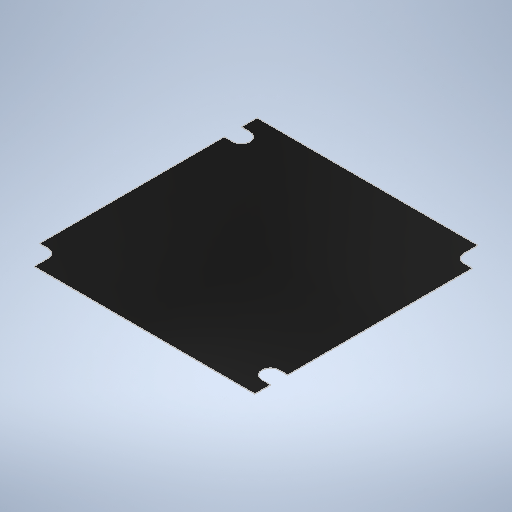
# Autodesk Inventor part: Coverplate Film
Saved by Autodesk Inventor 2025 (Build 290162000, 162)
## iProperties
Created: 2022-02-23
Part Number: Coverplate Film
Material: Thermoplastic Resin
Document SubType Name: Modeling
Designer: Caleb
Density: 1.28 g/cm^3
Appearance: Smooth - Black
Author: Caleb
Autodesk Inventor part; units mm, degrees
ref_plane "YZ Plane" through (0, 0, 0) normal (1, 0, 0) x (0, 1, 0)
ref_plane "XZ Plane" through (0, 0, 0) normal (0, 1, 0) x (-1, 0, 0)
ref_plane "XY Plane" through (0, 0, 0) normal (0, 0, 1) x (1, 0, 0)
sketch "Sketch1" plane through (0, 0, 0) normal (0, 1, 0) x (-1, 0, 0)
  line L0 (-20.8, -21) -> (20.8, -21)
  line L1 (20.8, -21) -> (20.8, 21)
  line L2 (20.8, 21) -> (-20.8, 21)
  line L3 (-20.8, 21) -> (-20.8, -21)
  line L4 (-20.8, -21) -> (20.8, 21) construction
  line L5 (20.8, -21) -> (-20.8, 21) construction
  point P0 (0, 0)
  dimension "d0" = 42
  dimension "d1" = 41.6
  constraints: 12 end point, 2 midpoint, 2 parallel, 1 horizontal, 1 perpendicular
  measures "d0" distance of L0.end L1.end
  measures "d1" distance of L1.end L2.end
extrude "Extrusion1" add sketch "Sketch1" along normal blind 0.08
sketch "Sketch2" plane through (0, 0.08, 0) normal (0, 1, 0) x (1, 0, 0)
  line L0 (-20.8, 21) -> (-20.8, -21) projected
  line L1 (-20.8, 18.3058) -> (-20.8, 15.1942)
  line L2 (-20.8, -17.05) -> (-20.8, -20.05)
  line L3 (20.8, 21) -> (-20.8, 21) projected
  line L4 (-22.3, 16.75) -> (-19.3, 16.75) construction
  line L5 (-22.3, 15.25) -> (-19.3, 15.25)
  line L6 (-19.3, 18.25) -> (-22.3, 18.25)
  arc A0 (-22.3, 18.25) -> (-22.3, 15.25) centre (-22.3, 16.75) ccw
  arc A1 (-19.3, 15.25) -> (-19.3, 18.25) centre (-19.3, 16.75) ccw
  line L7 (-22.3, -18.55) -> (-19.3, -18.55) construction
  line L8 (-22.3, -20.05) -> (-19.3, -20.05)
  line L9 (-19.3, -17.05) -> (-22.3, -17.05)
  arc A2 (-22.3, -17.05) -> (-22.3, -20.05) centre (-22.3, -18.55) ccw
  arc A3 (-19.3, -20.05) -> (-19.3, -17.05) centre (-19.3, -18.55) ccw
  line L10 (-20.8, -21) -> (20.8, -21) projected
  line L11 (20.8, -21) -> (20.8, 21) projected
  line L12 (22.3, -16.75) -> (19.3, -16.75) construction
  line L13 (22.3, -15.25) -> (19.3, -15.25)
  line L14 (20.8, -18.3058) -> (20.8, -15.1942)
  arc A4 (22.3, -18.25) -> (22.3, -15.25) centre (22.3, -16.75) ccw
  arc A5 (19.3, -15.25) -> (19.3, -18.25) centre (19.3, -16.75) ccw
  line L15 (19.3, -18.25) -> (22.3, -18.25)
  arc A6 (19.3, 20.05) -> (19.3, 17.05) centre (19.3, 18.55) ccw
  line L16 (19.3, 17.05) -> (22.3, 17.05)
  line L17 (20.8, 17.05) -> (20.8, 20.05)
  line L18 (22.3, 18.55) -> (19.3, 18.55) construction
  line L19 (22.3, 20.05) -> (19.3, 20.05)
  arc A7 (22.3, 17.05) -> (22.3, 20.05) centre (22.3, 18.55) ccw
  point P0 (-20.8, 16.75)
  point P1 (-20.8, 16.75)
  point P2 (-20.8, -18.55)
  point P3 (0, 0)
  point P4 (20.8, -16.75)
  point P5 (20.8, -16.75)
  point P6 (20.8, 18.55)
  point P7 (20.8, 17.05)
  point P8 (20.8, -18.25)
  point P9 (20.8, -15.25)
  point P10 (-20.8, 18.25)
  point P11 (-20.8, 15.25)
  dimension "d16" = 1.5
  dimension "d17" = 4.25
  dimension "d18" = 1.5
  dimension "d20" = 1.5
  dimension "d22" = 39.55
  dimension "d23" = 21
  dimension "d24" = 42
  dimension "d25" = 41.6
  dimension "d26" = 20.8
  dimension "d29" = 360
  constraints: 40 end point, 16 point on circle, 8 centre point, 8 tangent, 5 point on line, 3 midpoint, 2 collinear, 2 horizontal, 2 parallel, 1 horizontal alignment, 1 vertical alignment, 63 other
  measures "d16" radius of A1
  measures "d17" distance from line of L3 point (-20.8, 16.75)
  measures "d18" distance of L4.end point (-20.8, 16.75)
  measures "d20" radius of A3
  measures "d22" distance from line of L3 point (-20.8, -18.55)
  measures "d23" distance from line of L3 point (0, 0)
  measures "d24" distance between parallel lines of L3 L10
  measures "d25" distance of L0.end L10.end
  measures "d26" distance from line of point (0, 0) L11
extrude "Extrusion2" cut sketch "Sketch2" against normal blind 0.08 contours L6 A1 L5 L0 | L11 L16 A6 L19 | L9 A3 L8 L0 | L11 L15 A5 L13
sketch "Sketch3" plane through (0, 0.08, 0) normal (0, 1, 0) x (1, 0, 0)
  arc A0 (19.3, 20.05) -> (19.3, 17.05) centre (19.3, 18.55) ccw projected
  line L0 (17.8, 18.55) -> (17.8, 21)
  line L1 (20.8, 21) -> (-20.8, 21) projected
  line L2 (20.8, 20.05) -> (20.8, 21) projected
  line L3 (19.3, 20.05) -> (20.8, 20.05) projected
  line L4 (-19.3, -20.05) -> (-20.8, -20.05) projected
  arc A1 (-19.3, -20.05) -> (-19.3, -17.05) centre (-19.3, -18.55) ccw projected
  line L5 (-20.8, -20.05) -> (-20.8, -21) projected
  line L6 (-20.8, -21) -> (20.8, -21) projected
  line L7 (-17.8, -18.55) -> (-17.8, -21)
  point P0 (0, 0)
  constraints: 4 end point, 2 point on circle, 2 point on line, 1 horizontal alignment, 1 perpendicular, 1 vertical
extrude "Extrusion3" cut sketch "Sketch3" against normal blind 0.08
equation "\"d20\" = d16"
equation "\"d23\" = 0.5 * d24"
equation "\"d26\" = 0.5 * d25"
body "Solid1"
